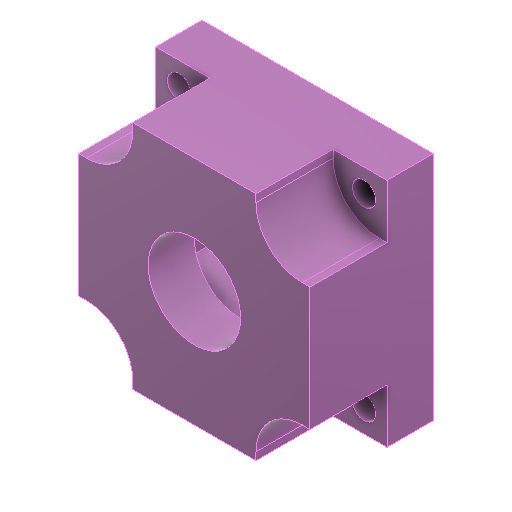
# Autodesk Inventor part: sujecion_cable
Saved by Autodesk Inventor 2026.1 (Build 301233000, 233)
## iProperties
Created: 2025-10-01
Part Number: sujecion_cable
Material: Genérico
Document SubType Name: Modeling
Designer: gianm
Density: 1 g/cm^3
Appearance: Suave - Púrpura
Author: gianm
Autodesk Inventor part; units mm, degrees
ref_plane "YZ Plane" through (0, 0, 0) normal (1, 0, 0) x (0, 1, 0)
ref_plane "XZ Plane" through (0, 0, 0) normal (0, 1, 0) x (-1, 0, 0)
ref_plane "XY Plane" through (0, 0, 0) normal (0, 0, 1) x (1, 0, 0)
sketch "Boceto1" plane through (0, 0, 0) normal (0, 0, 1) x (1, 0, 0)
  line L0 (-7.5, -7.5) -> (7.5, -7.5)
  line L1 (7.5, -7.5) -> (7.5, 7.5)
  line L2 (7.5, 7.5) -> (-7.5, 7.5)
  line L3 (-7.5, 7.5) -> (-7.5, -7.5)
  line L4 (-7.5, -7.5) -> (7.5, 7.5) construction
  line L5 (7.5, -7.5) -> (-7.5, 7.5) construction
  dimension "d2" = 15
  constraints: 12 end point, 2 parallel, 2 perpendicular, 1 horizontal
  measures "d2" distance of L1.end L2.end
extrude "Extrusión1" add sketch "Boceto1" against normal blind 8
sketch "Boceto2" plane through (0, 0, -8) normal (0, 0, -1) x (-1, 0, 0)
  circle A0 centre (-6, 6) radius 0.75
  line L0 (6, -6) -> (-6, -6) construction
  line L1 (-6, -6) -> (-6, 6) construction
  line L2 (-6, 6) -> (6, 6) construction
  line L3 (6, 6) -> (6, -6) construction
  line L4 (6, -6) -> (-6, 6) construction
  line L5 (-6, -6) -> (6, 6) construction
  circle A1 centre (6, 6) radius 0.75
  circle A2 centre (6, -6) radius 0.75
  circle A3 centre (-6, -6) radius 0.75
  point P0 (0, 0)
  dimension "d5" = 12
  dimension "d6" = 1.5
  constraints: 12 end point, 4 centre point, 3 coincident, 3 equal radius, 2 midpoint, 2 parallel, 2 perpendicular, 1 horizontal
  measures "d5" distance of L1.end L2.end
  measures "d6" diameter of A1
extrude "Extrusión2" cut sketch "Boceto2" against normal up to surface (8 mm away)
sketch "Boceto3" plane through (0, 0, 0) normal (0, 0, 1) x (1, 0, 0)
  line L0 (7.5, 7.5) -> (-7.5, 7.5) projected
  line L1 (-7.5, 7.5) -> (-4, 7.5)
  line L2 (-4, 7.5) -> (-4, 4)
  line L3 (-4, 4) -> (-7.5, 4)
  line L4 (-7.5, 4) -> (-7.5, 7.5)
  line L5 (-7.5, -7.5) -> (-7.5, -4)
  line L6 (-7.5, -4) -> (-4, -4)
  line L7 (-4, -4) -> (-4, -7.5)
  line L8 (-4, -7.5) -> (-7.5, -7.5)
  line L9 (7.5, -7.5) -> (4, -7.5)
  line L10 (4, -7.5) -> (4, -4)
  line L11 (4, -4) -> (7.5, -4)
  line L12 (7.5, -4) -> (7.5, -7.5)
  line L13 (7.5, 7.5) -> (7.5, 4)
  line L14 (7.5, 4) -> (4, 4)
  line L15 (4, 4) -> (4, 7.5)
  line L16 (4, 7.5) -> (7.5, 7.5)
  point P0 (0, 0)
  point P1 (0, 0)
  point P2 (0, 0)
  point P3 (0, 0)
  dimension "d9" = 3.5
  dimension "d12" = 360
  constraints: 32 end point, 2 coincident, 2 parallel, 1 horizontal, 1 perpendicular, 35 other
  measures "d9" distance of L2.end L3.end
extrude "Extrusión3" cut sketch "Boceto3" against normal blind 5
fillet "Empalme1" radius 3 4 edges at (-4, 4, -2.5) (4, 4, -2.5) (4, -4, -2.5) (-4, -4, -2.5)
sketch "Boceto4" plane through (0, 0, -8) normal (0, 0, -1) x (-1, 0, 0)
  line L0 (0, 5.7735) -> (5, 2.8868)
  line L1 (5, 2.8868) -> (5, -2.8868)
  line L2 (5, -2.8868) -> (0, -5.7735)
  line L3 (0, -5.7735) -> (-5, -2.8868)
  line L4 (-5, -2.8868) -> (-5, 2.8868)
  line L5 (-5, 2.8868) -> (0, 5.7735)
  point P0 (0, 0)
  point P1 (0, 0)
  dimension "d17" = 10
  constraints: 12 end point, 1 coincident, 13 other
  measures "d17" distance between parallel lines of L2 L5
extrude "Extrusión4" cut sketch "Boceto4" against normal blind 5
sketch "Boceto5" plane through (0, 0, 0) normal (0, 0, 1) x (1, 0, 0)
  circle A0 centre (0, 0) radius 3
  dimension "d20" = 6
  constraints: 1 centre point, 1 coincident
  measures "d20" diameter of A0
extrude "Extrusión5" cut sketch "Boceto5" against normal up to surface (8 mm away)
